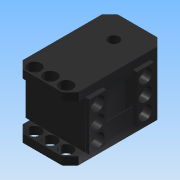
# Autodesk Inventor part: Motor
Saved by Autodesk Inventor 2015 (Build 190159000, 159)
## iProperties
Created: 2014-03-07
Part Number: Motor
Material: Générique
Document SubType Name: Modeling
Designer: Grégoire
Density: 1 g/cm^3
Appearance: Par défaut
Author: Grégoire
Autodesk Inventor part; units mm, degrees
ref_plane "YZ Plane" through (0, 0, 0) normal (1, 0, 0) x (0, 1, 0)
ref_plane "XZ Plane" through (0, 0, 0) normal (0, 1, 0) x (-1, 0, 0)
ref_plane "XY Plane" through (0, 0, 0) normal (0, 0, 1) x (1, 0, 0)
sketch "Esquisse2" plane through (0, 0, 0) normal (0, 0, 1) x (1, 0, 0)
  line L0 (0, 0) -> (15, 0)
  line L1 (18, 3) -> (18, 33)
  line L2 (15, 36) -> (0, 36)
  line L3 (-3, 33) -> (-3, 3)
  line L4 (-3, 3) -> (0, 0)
  line L5 (0, 36) -> (-3, 33)
  line L6 (15, 36) -> (18, 33)
  line L7 (18, 3) -> (15, 0)
  line L8 (0, 36) -> (0, 0) construction
  line L9 (15, 0) -> (15, 36) construction
  line L10 (18, 33) -> (-3, 33) construction
  line L11 (18, 3) -> (-3, 3) construction
  dimension "d12" = 15
  dimension "d14" = 21
  dimension "d15" = 36
  constraints: 24 end point, 5 equal length, 3 perpendicular, 2 parallel, 1 coincident, 1 horizontal
  measures "d12" distance of L2.start L2.end
  measures "d14" distance between parallel lines of L1 L3
  measures "d15" distance between parallel lines of L2 L0
extrude "Extrusion1" add sketch "Esquisse2" along normal blind 24
sketch "Esquisse3" plane through (-3, 3, 0) normal (-1, 0, 0) x (0, 0, 1)
  line L0 (0, 0) -> (0, 30) construction
  line L1 (24, 30) -> (24, 0) construction
  line L2 (0, -3) -> (24, -3) construction
  line L3 (3, -3) -> (21, -3)
  line L4 (21, -3) -> (21, 2.6)
  line L5 (21, 2.6) -> (3, 2.6)
  line L6 (3, 2.6) -> (3, -3)
  line L7 (3, 2.6) -> (0, 2.6) construction
  line L8 (21, 2.6) -> (24, 2.6) construction
  dimension "d24" = 3
  dimension "d25" = 5.6
  constraints: 12 end point, 3 equal length, 3 point on line, 2 perpendicular, 1 collinear, 1 horizontal
  measures "d24" distance of L5.end L7.end
  measures "d25" distance of L3.end L4.end
extrude "Extrusion2" cut sketch "Esquisse3" against normal through all
sketch "Esquisse4" plane through (0, 0, 0) normal (0, 0, -1) x (-1, 0, 0)
  line L0 (-15, 0) -> (0, 0) construction
  line L1 (0, 0) -> (3, 3) construction
  line L2 (0, 36) -> (-15, 36) construction
  circle A0 centre (-7.5, 3) radius 2.5
  line L3 (-15, 0) -> (-7.5, 3) construction
  line L4 (0, 0) -> (-7.5, 3) construction
  line L5 (-7.5, 3) -> (3, 3) construction
  circle A1 centre (-1.5, 3) radius 2.5
  circle A2 centre (-13.5, 3) radius 2.5
  circle A3 centre (-7.5, 3) radius 2.5
  dimension "d28" = 0.5
  dimension "d29" = 5
  dimension "d32" = 6
  dimension "d35" = 6
  constraints: 6 end point, 4 centre point, 2 horizontal, 1 equal length, 1 parallel, 1 point on line, 6 other
  measures "d28" distance edge to line of A0 L0
  measures "d29" diameter of A0
  measures "d32" distance of L3.end A1.centre
  measures "d35" distance of L3.end A2.centre
extrude "Extrusion3" cut sketch "Esquisse4" against normal through all
sketch "Esquisse5" plane through (0, 0, 0) normal (0, 0, -1) x (-1, 0, 0)
  circle A0 centre (-7.5, 3) radius 2.5 construction
  line L0 (3, 3) -> (3, 33) construction
  line L1 (0, 36) -> (-15, 36) construction
  line L2 (-7.5, 3) -> (-7.5, 36) construction
  circle A1 centre (-7.5, 27) radius 2.5
  line L3 (-7.5, 27) -> (3, 27) construction
  circle A2 centre (-1.5, 27) radius 2.5
  circle A3 centre (-13.5, 27) radius 2.5
  circle A4 centre (-7.5, 27) radius 2.5
  dimension "d40" = 5
  dimension "d41" = 24
  dimension "d44" = 6
  dimension "d47" = 6
  constraints: 4 centre point, 4 end point, 2 horizontal, 2 point on line, 1 midpoint, 1 perpendicular, 6 other
  measures "d40" diameter of A1
  measures "d41" distance of L2.start L3.start
  measures "d44" distance of L3.start A2.centre
  measures "d47" distance of L3.start A3.centre
extrude "Extrusion4" cut sketch "Esquisse5" against normal blind 3
sketch "Esquisse7" plane through (7.5, 27, 3) normal (0, 0, -1) x (-1, 0, 0)
  circle A0 centre (0, 0) radius 2.5 projected
  circle A1 centre (0, 0) radius 2
  point P0 (7.5, -27)
  dimension "d54" = 4
  constraints: 1 centre point, 1 coincident
  measures "d54" diameter of A1
extrude "Extrusion6" cut sketch "Esquisse7" against normal through all contours A1
sketch "Esquisse8" plane through (18, 3, 0) normal (1, 0, 0) x (0, 0, -1)
  line L0 (0, 30) -> (0, 0) construction
  line L1 (0, 26.5) -> (0, 21.5) projected
  line L2 (-24, 21.4697) -> (-24, 26.4697) projected
  line L3 (-24, 23.9697) -> (0, 24) construction
  line L4 (-21, 20.7349) -> (-3, 20.7349)
  line L5 (-3, 20.7349) -> (-3, 27.2349)
  line L6 (-3, 27.2349) -> (-21, 27.2349)
  line L7 (-21, 27.2349) -> (-21, 20.7349)
  line L8 (-21, 20.7349) -> (-3, 27.2349) construction
  line L9 (-3, 20.7349) -> (-21, 27.2349) construction
  line L10 (-21, 2.6) -> (-3, 2.6) projected
  line L11 (-12, 23.9849) -> (-12, 2.6) construction
  line L12 (-21, 2.7349) -> (-3, 2.7349)
  line L13 (-3, 2.7349) -> (-3, 9.2349)
  line L14 (-3, 9.2349) -> (-21, 9.2349)
  line L15 (-21, 9.2349) -> (-21, 2.7349)
  point P0 (0, -3)
  dimension "d57" = 6.5
  dimension "d58" = 18
  dimension "d74" = 18
  constraints: 24 end point, 6 midpoint, 2 parallel, 1 horizontal, 1 perpendicular, 1 vertical, 8 other
  measures "d57" distance of L6.end L4.start
  measures "d58" distance of L5.end L6.end
  measures "d74" distance of L4.start L12.start
extrude "Extrusion7" add sketch "Esquisse8" along normal blind 1.5
sketch "Esquisse9" plane through (19.5, 3, 0) normal (1, 0, 0) x (0, 0, -1)
  line L0 (-3, 20.7349) -> (-3, 27.2349) construction
  line L1 (-21, 27.2349) -> (-21, 20.7349) construction
  line L2 (-21, 23.9849) -> (-3, 23.9849) construction
  circle A0 centre (-12, 23.9849) radius 2.5
  line L3 (-15, 23.9849) -> (3, 23.9849) construction
  circle A1 centre (-6, 23.9849) radius 2.5
  line L4 (-27, 23.9849) -> (-9, 23.9849) construction
  circle A2 centre (-18, 23.9849) radius 2.5
  line L5 (-21, 23.9849) -> (-3, 23.9849) construction
  circle A3 centre (-12, 23.9849) radius 2.5
  line L6 (-21, 20.7349) -> (-3, 20.7349) projected
  line L7 (-12, 23.9849) -> (-12, 11.4292) construction
  circle A4 centre (-12, 5.9849) radius 2.5
  circle A5 centre (-6, 5.9849) radius 2.5
  circle A6 centre (-18, 5.9849) radius 2.5
  point P0 (0, -3)
  dimension "d61" = 5
  dimension "d64" = 6
  dimension "d67" = 6
  dimension "d81" = 18
  constraints: 10 end point, 7 centre point, 3 midpoint, 2 collinear, 2 horizontal, 1 perpendicular, 1 vertical, 19 other
  measures "d61" diameter of A0
  measures "d64" distance of L2.start L3.start
  measures "d67" distance of L2.start L4.start
  measures "d81" distance of A2.centre A6.centre
extrude "Extrusion8" cut sketch "Esquisse9" against normal blind 3
sketch "Esquisse10" plane through (-3, 3, 0) normal (-1, 0, 0) x (0, 0, 1)
  line L0 (3, 27.2349) -> (21, 27.2349) projected
  line L1 (21, 27.2349) -> (21, 20.7349) projected
  line L2 (21, 20.7349) -> (3, 20.7349) projected
  line L3 (3, 20.7349) -> (3, 27.2349) projected
  line L4 (21, 9.2349) -> (21, 2.7349) projected
  line L5 (21, 2.7349) -> (3, 2.7349) projected
  line L6 (3, 2.7349) -> (3, 9.2349) projected
  line L7 (3, 9.2349) -> (21, 9.2349) projected
  point P0 (0, -3)
extrude "Extrusion9" add sketch "Esquisse10" along normal blind 1.5
sketch "Esquisse11" plane through (-4.5, 3, 0) normal (-1, 0, 0) x (0, 0, 1)
  circle A0 centre (6, 23.9849) radius 2.5 projected
  circle A1 centre (12, 23.9849) radius 2.5 projected
  circle A2 centre (18, 23.9849) radius 2.5 projected
  circle A3 centre (18, 5.9849) radius 2.5 projected
  circle A4 centre (12, 5.9849) radius 2.5 projected
  circle A5 centre (6, 5.9849) radius 2.5 projected
  point P0 (0, -3)
extrude "Extrusion10" cut sketch "Esquisse11" against normal blind 1.5
sketch "Esquisse13" plane through (18, 3, 0) normal (1, 0, 0) x (0, 0, -1)
  line L0 (-21, 9.2349) -> (-3, 9.2349) projected
  line L1 (-3, 20.7349) -> (-18.5, 20.7349)
  line L2 (-18.5, 20.7349) -> (-18.5, 9.2349)
  line L3 (-18.5, 9.2349) -> (-3, 9.2349)
  line L4 (-3, 9.2349) -> (-3, 20.7349)
  point P0 (0, -3)
  dimension "d90" = 15.5
  constraints: 8 end point, 2 parallel, 1 horizontal, 1 perpendicular, 1 point on line
  measures "d90" distance between parallel lines of L4 L2
extrude "Extrusion11" cut sketch "Esquisse13" against normal blind 3
sketch "Esquisse14" plane through (18, 3, 0) normal (1, 0, 0) x (0, 0, -1)
  line L0 (-21, 20.7349) -> (-3, 20.7349) projected
  line L1 (-3, 9.2349) -> (-21, 9.2349) projected
  line L2 (-3, 20.7349) -> (-9, 20.7349)
  line L3 (-9, 20.7349) -> (-9, 9.2349)
  line L4 (-9, 9.2349) -> (-3, 9.2349)
  line L5 (-3, 9.2349) -> (-3, 20.7349)
  point P0 (0, -3)
  dimension "d93" = 6
  constraints: 8 end point, 2 parallel, 1 horizontal, 1 perpendicular, 1 point on line
  measures "d93" distance between parallel lines of L5 L3
extrude "Extrusion12" add sketch "Esquisse14" against normal blind 0.2
sketch "Esquisse16" plane through (-3, 3, 0) normal (-1, 0, 0) x (0, 0, 1)
  line L0 (3, 9.2349) -> (21, 9.2349) construction
  line L1 (3, 20.7349) -> (18.5, 20.7349)
  line L2 (18.5, 20.7349) -> (18.5, 9.2349)
  line L3 (18.5, 9.2349) -> (3, 9.2349)
  line L4 (3, 9.2349) -> (3, 20.7349)
  point P0 (0, -3)
  dimension "d96" = 15.5
  constraints: 8 end point, 2 parallel, 1 horizontal, 1 perpendicular, 1 point on line
  measures "d96" distance between parallel lines of L2 L4
extrude "Extrusion13" cut sketch "Esquisse16" against normal blind 3
sketch "Esquisse17" plane through (-3, 3, 0) normal (-1, 0, 0) x (0, 0, 1)
  line L0 (3, 20.7349) -> (9, 20.7349)
  line L1 (9, 20.7349) -> (9, 9.2197)
  line L2 (9, 9.2197) -> (3, 9.2197)
  line L3 (3, 9.2197) -> (3, 20.7349)
  line L4 (3, 9.2349) -> (3, 20.7349) projected
  point P0 (0, -3)
  dimension "d99" = 6
  constraints: 8 end point, 2 parallel, 1 horizontal, 1 perpendicular
  measures "d99" distance between parallel lines of L4 L1
extrude "Extrusion14" add sketch "Esquisse17" against normal blind 0.2
fillet "Congé1" radius 1 9 edges at (18, 33, 12) (15, 36, 12) (0, 36, 12) (0, 0, 1.5) (0, 0, 22.5) (15, 0, 1.5) (18, 3, 1.5) (15, 0, 22.5) (18, 3, 22.5)
chamfer "Chanfrein1" distance 0.5 angle 45 2 edges at (-3, 17.9849, 18.5) (18, 17.9849, 18.5)
